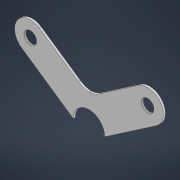
# Autodesk Inventor part: FixaçãoTanque_1
Saved by Autodesk Inventor 2022 (Build 260153000, 153)
## iProperties
Created: 2022-05-19
Part Number: FixaçãoTanque_1
Material: Genérico
Document SubType Name: Modeling
Designer: Gugarauj07
Density: 1 g/cm^3
Appearance: Padrão
Author: Gugarauj07
Autodesk Inventor part; units mm, degrees
ref_plane "YZ Plane" through (0, 0, 0) normal (1, 0, 0) x (0, 1, 0)
ref_plane "XZ Plane" through (0, 0, 0) normal (0, 1, 0) x (-1, 0, 0)
ref_plane "XY Plane" through (0, 0, 0) normal (0, 0, 1) x (1, 0, 0)
sketch "Esboço1" plane through (0, 0, 0) normal (0, 0, 1) x (1, 0, 0)
  arc A0 (0, 12.7) -> (-12.7, 0) centre (0, 0) ccw
  line L0 (-12.7, 0) -> (-54.5577, 28.729)
  arc A1 (-40.1843, 49.671) -> (-54.5577, 28.729) centre (-47.371, 39.2) ccw
  line L1 (-40.1843, 49.671) -> (-8.5885, 27.9852)
  circle A2 centre (-47.371, 39.2) radius 5.08
  line L2 (0, 0) -> (0, 58.6538)
  arc A3 (12.7, 0) -> (0, 12.7) centre (0, 0) ccw
  line L3 (12.7, 0) -> (54.5577, 28.729)
  arc A4 (54.5577, 28.729) -> (40.1843, 49.671) centre (47.371, 39.2) ccw
  line L4 (40.1843, 49.671) -> (8.5885, 27.9852)
  circle A5 centre (47.371, 39.2) radius 5.08
  arc A6 (-8.5885, 27.9852) -> (0, 24.8739) centre (1.2712, 41.7925) ccw
  arc A7 (0, 24.8739) -> (8.5885, 27.9852) centre (-1.2712, 41.7925) ccw
  point P0 (0, 25.2951)
  dimension "d2" = 12.7
  dimension "d3" = 10.16
  dimension "d4" = 94.742
  dimension "d5" = 39.2
  dimension "d6" = 12.7
  dimension "d7" = 55.536
  dimension "d9" = 9
  dimension "d10" = 25.4
  dimension "d11" = 111.073
  dimension "d14" = 50.7684
  dimension "d15" = 25.4
  constraints: 12 point on circle, 10 end point, 8 centre point, 7 symmetric about line, 3 coincident, 2 point on line, 1 parallel, 1 tangent, 1 vertical, 7 other
  measures "d2" radius of A1
  measures "d3" diameter of A2
  measures "d4" diameter of A1.centre L2
  measures "d5" vertical distance of L0.start A1.centre
  measures "d6" radius of A0
  measures "d7" angle of L2 L1
  measures "d9" distance of L1.end point (0, 25.295)
  measures "d10" distance of L3.start L0.start
  measures "d11" angle of L4 L1
  measures "d14" distance of L0.start L0.end
  measures "d15" distance between parallel lines of L3 L4
extrude "Extrusão1" add sketch "Esboço1" along normal blind 1.6
